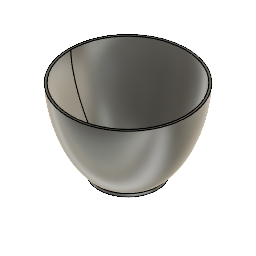
lampshade (Autodesk Fusion 360 design; units mm, degrees)
Autodesk Fusion 360 part; units mm, degrees
sketch "Sketch1" plane through (0, 0, 0) normal (0, 1, 0) x (1, 0, 0)
  line L0 (-0.0536, -61.5771) -> (-0.0536, 35.4229) construction
  spline S0 degree 5 poles (-28.0536, -36.939) (-28.0663, -35.7869) (-27.9746, -33.3482) (-27.4866, -29.2872) (-26.1883, -23.2234) (-23.5413, -15.2455) (-20.4715, -9.1418) (-17.4725, -5.0243) (-15.1228, -2.5348) (-13.8603, -1.354) knots 0 0 0 0 0 0 0.2 0.4 0.6 0.8 1 1 1 1 1 1
  line L1 (-27.9987, -41.939) -> (-28.1085, -31.939)
  line L2 (-19.2881, -6.4304) -> (-8.4326, 3.7224)
  line L3 (-13.8603, -1.354) -> (-13.8603, 0.061)
  line L4 (-13.8603, 0.061) -> (-11.6214, 0.061)
  line L5 (-11.6214, 0.061) -> (-10.6214, -0.5757)
  line L6 (-10.6214, -0.5757) -> (-10.6214, -1.2207)
  line L7 (-11.5536, -1.8425) -> (-11.5536, -2.0689)
  spline S1 degree 5 poles (-27.0536, -36.939) (-27.0536, -35.7848) (-26.9154, -33.3535) (-26.2936, -29.3379) (-24.715, -23.3918) (-21.6612, -15.6099) (-18.3217, -9.6652) (-15.204, -5.6516) (-12.8212, -3.222) (-11.5536, -2.0689) knots 0 0 0 0 0 0 0.2 0.4 0.6 0.8 1 1 1 1 1 1
  line L8 (-27.0537, -41.9415) -> (-27.0536, -31.9365)
  line L9 (-17.0518, -7.0709) -> (-6.0555, 2.9332)
  line L10 (-28.0536, -36.939) -> (-27.0536, -36.939)
  line L11 (-11.5536, -1.8425) -> (-10.6214, -1.2207)
  dimension "d7" = 37
  dimension "d8" = 11.5
  dimension "d9" = 27
  dimension "d10" = 1
  dimension "d11" = 1
  dimension "d12" = 3.2389
  dimension "d13" = 2.3067
  measures "d7" distance of S0.start L4
  measures "d8" distance of L0 L7
  measures "d9" distance of L0 S1.start
  measures "d10" distance of S0.start S1.start
  measures "d11" distance of L4.end L6
  measures "d12" distance of L3 L6
  measures "d13" distance of S0.end L7.end
revolve "Revolve1" add sketch "Sketch1" angle 360 about axis through (-0.0536, 0, 61.5771) along (0, 0, -1) contours S0 L2 L4 L5 L6 L7 S1 L10 L11 | L2 L3 L4
